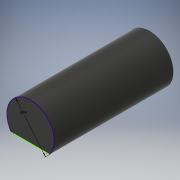
# Autodesk Inventor part: DPLX_P026_VIPE _Transformer
Saved by Autodesk Inventor 2018 (Build 220112000, 112)
## iProperties
Created: 2017-09-30
Part Number: DPLX_P026_VIPE _Transformer
Material: PC/ABS Plastic
Document SubType Name: Modeling
Designer: Sam
Density: 0.357273 g/cm^3
Appearance: Fine Textured - Black
Mass: 9.3516 g
Surface Area: 76.7492 cm^2
Volume: 26.175 cm^3
Author: Sam
Autodesk Inventor part; units mm, degrees
ref_plane "YZ Plane" through (0, 0, 0) normal (1, 0, 0) x (0, 1, 0)
ref_plane "XZ Plane" through (0, 0, 0) normal (0, 1, 0) x (-1, 0, 0)
ref_plane "XY Plane" through (0, 0, 0) normal (0, 0, 1) x (1, 0, 0)
sketch "Sketch1" plane through (0, 0, 0) normal (0, 0, 1) x (1, 0, 0)
  arc A0 (10.1214, -7.3299) -> (-10.1214, -7.3299) centre (0, 0) ccw
  line L0 (-10.1214, -7.3299) -> (10.1214, -7.3299)
  dimension "d0" = 24.9936
  constraints: 2 end point, 2 point on circle, 1 centre point, 1 coincident, 1 horizontal
  measures "d0" diameter of A0
extrude "Extrusion1" add sketch "Sketch1" along normal blind 63
sketch "Sketch4" plane through (0, 0, 63) normal (0, 0, 1) x (1, 0, 0)
  arc A0 (10.1214, -7.3299) -> (-10.1214, -7.3299) centre (0, 0) ccw
  line L0 (-10.1214, -7.3299) -> (10.1214, -7.3299)
  line L1 (-10.1214, -7.3299) -> (10.1214, -7.3299) projected
  point P0 (-8.8613, -7.3299)
  point P1 (8.8613, -7.3299)
  dimension "d8" = 24.9936
  constraints: 2 end point, 2 point on circle, 1 centre point, 1 coincident, 1 collinear
  measures "d8" diameter of A0
